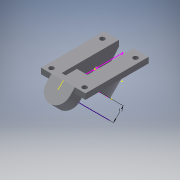
# Autodesk Inventor part: shaft_jig
Saved by Autodesk Inventor 2017 SP1 (Build 210196100, 196)
## iProperties
Part Number: shaft_jig
Material: 一般
Document SubType Name: Modeling
Designer: gisen
Density: 1 g/cm^3
Appearance: 既定
Author: gisen
Autodesk Inventor part; units mm, degrees
ref_plane "YZ Plane" through (0, 0, 0) normal (1, 0, 0) x (0, 1, 0)
ref_plane "XZ Plane" through (0, 0, 0) normal (0, 1, 0) x (-1, 0, 0)
ref_plane "XY Plane" through (0, 0, 0) normal (0, 0, 1) x (1, 0, 0)
sketch "スケッチ1" plane through (0, 0, 0) normal (0, 0, 1) x (1, 0, 0)
  line L0 (-27.5, -39) -> (27.5, -39)
  line L1 (27.5, -39) -> (27.5, 39)
  line L2 (27.5, 39) -> (-27.5, 39)
  line L3 (-27.5, 39) -> (-27.5, -39)
  line L4 (-27.5, -39) -> (27.5, 39) construction
  line L5 (27.5, -39) -> (-27.5, 39) construction
  point P0 (0, 0)
  dimension "d0" = 55
  dimension "d1" = 78
  constraints: 12 end point, 2 midpoint, 2 parallel, 1 horizontal, 1 perpendicular
  measures "d0" distance of L2.end L1.end
  measures "d1" distance of L1.end L0.end
extrude "押し出し1" add sketch "スケッチ1" along normal blind 7
sketch "スケッチ2" plane through (0, 0, 7) normal (0, 0, 1) x (1, 0, 0)
  line L0 (9, -27) -> (9, 39)
  line L1 (9, 39) -> (-9, 39)
  line L2 (-9, 39) -> (-9, -27)
  line L3 (-9, -27) -> (9, -27)
  line L4 (9, -27) -> (-9, 39) construction
  line L5 (9, 39) -> (-9, -27) construction
  point P0 (0, 0)
  point P1 (0, 6)
  dimension "d4" = 18
  dimension "d5" = 66
  dimension "d15" = 9
  constraints: 12 end point, 2 midpoint, 2 parallel, 1 perpendicular
  measures "d4" distance of L1.end L0.end
  measures "d5" distance of L0.start L0.end
  measures "d15" distance from line of L0 point (0, 0)
extrude "押し出し2" cut sketch "スケッチ2" against normal blind 7
ref_plane "作業平面1" through (-27.5, -39, 7) normal (0, 0.7071068, -0.7071068) x (1, 0, 0)
sketch "スケッチ5" plane through (-27.5, -39, 7) normal (0, 0.7071068, -0.7071068) x (1, 0, 0)
  line L0 (0, 4.9497) -> (55, 4.9497) projected
  line L1 (55, 4.9497) -> (55, 0) projected
  line L2 (0, 0) -> (55, 0) projected
  line L3 (0, 4.9497) -> (0, 0) projected
  line L4 (27.5, 9) -> (42, 9) construction
  line L5 (27.5, 9) -> (42, 9) construction
  line L6 (27.5, 9) -> (13, 9) construction
  line L7 (42, 0) -> (13, 0)
  line L8 (13, 0) -> (13, 9)
  line L9 (42, 9) -> (42, 0)
  line L10 (42, 9) -> (13, 9)
  line L11 (13, 9) -> (13, 0)
  line L12 (13, 0) -> (42, 0)
  line L13 (42, 0) -> (42, 9)
  arc A0 (42, 9) -> (13, 9) centre (27.5, 9) ccw
  point P0 (27.5, -22.6274)
  dimension "d14" = 180
  dimension "d16" = 9
  dimension "d17" = 0
  dimension "d18" = 9
  dimension "d19" = 55
  dimension "d20" = 27.5
  constraints: 20 end point, 2 horizontal, 2 parallel, 2 perpendicular, 2 point on circle, 1 centre point, 1 coincident, 1 collinear, 1 vertical
  measures "d14" angle of L6 L4
  measures "d16" distance of L5.end L7.start
  measures "d17" distance between parallel lines of L7 L2
  measures "d18" distance of L7.end L6.end
  measures "d19" distance of L0.start L0.end
  measures "d20" distance from line of L3 L4.start
extrude "押し出し4" add sketch "スケッチ5" along normal blind 17 contours L8 L10 L9 L0 | L0 L9 L2 L8 | A0 L10
sketch "スケッチ6" plane through (-14.5, -26.9792, -5.0208) normal (0, 0.7071068, 0.7071068) x (1, 0, 0)
  line L0 (5.5, -7.1005) -> (23.5, -7.1005) projected
  line L1 (29, -7.1005) -> (0, -7.1005) projected
  line L2 (29, -7.1005) -> (29, 0) projected
  line L3 (0, 0) -> (29, 0) projected
  line L4 (0, -7.1005) -> (0, 0) projected
  line L5 (0, -17) -> (0, 0) projected
  line L6 (29, -7.1005) -> (0, -7.1005)
  line L7 (0, -7.1005) -> (0, 0)
  line L8 (0, 0) -> (29, 0)
  line L9 (29, 0) -> (29, -7.1005)
  point P0 (14.5, 15.5269)
  constraints: 8 end point, 2 parallel, 1 horizontal, 1 perpendicular
extrude "押し出し5" add sketch "スケッチ6" along normal up to surface surface through (0, 0, 0) normal (0, 0, 1)
chamfer "面取り1" distance 5 angle 45 1 edges at (0, -27, 7)
sketch "スケッチ8" plane through (-9, -21.9584, 0) normal (0, 0, 1) x (1, 0, 0)
  line L0 (18, -5.0416) -> (18, 0) projected
  line L1 (0, 0) -> (18, 0) projected
  line L2 (0, 0) -> (0, -5.0416) projected
  line L3 (0, -5.0416) -> (18, -5.0416) projected
  line L4 (0, -5.0416) -> (18, -5.0416) projected
  line L5 (0, -5.0416) -> (18, -5.0416)
  line L6 (18, -5.0416) -> (18, 8.9584)
  line L7 (18, 8.9584) -> (0, 8.9584)
  line L8 (0, 8.9584) -> (0, -5.0416)
  point P0 (9, 21.9584)
  dimension "d30" = 14
  constraints: 8 end point, 2 parallel, 1 horizontal, 1 perpendicular
  measures "d30" distance of L6.end L5.end
extrude "押し出し8" add sketch "スケッチ8" along normal blind 2
ref_plane "作業平面2" through (-27.5, 1.3051, -33.3051) normal (0, 0.7071068, -0.7071068) x (-1, 0, 0)
ref_plane "作業平面3" through (7.25, -21.9584, 0) normal (0, 0.7071068, 0.7071068) x (1, 0, 0)
sketch "スケッチ9" plane through (7.25, -21.9584, 0) normal (0, 0.7071068, 0.7071068) x (1, 0, 0)
  line L0 (-21.75, 0) -> (-21.75, -12.0503) projected
  line L1 (-34.75, -12.0503) -> (-21.75, -12.0503) projected
  line L2 (-34.75, 43.1041) -> (-34.75, -12.0503) projected
  line L3 (-16.25, 43.1041) -> (-34.75, 43.1041) projected
  line L4 (-16.25, 43.1041) -> (-16.25, 6.3345) projected
  line L5 (1.75, 6.3345) -> (-16.25, 6.3345) construction
  line L6 (1.75, 6.3345) -> (1.75, 43.1041) projected
  line L7 (20.25, 43.1041) -> (1.75, 43.1041) projected
  line L8 (20.25, -12.0503) -> (20.25, 43.1041) projected
  line L9 (7.25, -12.0503) -> (20.25, -12.0503) projected
  line L10 (7.25, -12.0503) -> (7.25, 0) projected
  line L11 (-21.75, 0) -> (7.25, 0) projected
  line L12 (-7.25, 40) -> (7.75, 40) construction
  line L13 (-7.25, 40) -> (7.75, 40) construction
  line L14 (-7.25, 40) -> (-7.25, 51.8983) construction
  line L15 (7.25, 0) -> (-21.75, 0) projected
  line L16 (7.75, 40) -> (7.75, 0)
  line L17 (7.75, 0) -> (-22.25, 0)
  line L18 (-22.25, 0) -> (7.75, 0)
  circle A0 centre (-7.25, 40) radius 4.5 projected
  circle A1 centre (-7.25, 40) radius 11 projected
  spline S0 degree 2 poles (-7.25, 50) (-26.3864, 48.3359) (-22.25, 0) knots 0 0 0 1 1 1
  line L19 (-7.25, 40) -> (-7.25, 50)
  spline S1 degree 2 poles (-7.25, 50) (11.8864, 48.3359) (7.75, 0) knots 0 0 0 1 1 1
  point P0 (-7.25, 15.5269)
  point P1 (-17.8029, 43.1041)
  point P2 (3.3029, 43.1041)
  dimension "d103" = 15
  dimension "d106" = 10
  constraints: 14 end point, 3 point on line, 2 coincident, 2 collinear, 1 horizontal, 1 perpendicular, 1 symmetric about line, 1 vertical, 8 other
  measures "d103" distance from line of L16 L12.start
  measures "d106" distance of L12.start L19.end
extrude "押し出し9" add sketch "スケッチ9" along normal up to surface contours L17 S0 A1 S1 L16 L11 | L16 S1 | S0 S1 L7 L6 A1 L4 L3 | L3 L4 A1 | A1 L6 L7 surface through (0, 0, 0) normal (0, 0, 1)
ref_plane "作業平面4" through (9, -13, 2) normal (0, 0.7071068, 0.7071068) x (-1, 0, 0)
sketch "スケッチ13" plane through (0, 0, 0) normal (1, 0, 0) x (0, 1, 0)
  line L0 (39, 0) -> (39, 7) projected
  line L1 (39, 0) -> (26.8843, -21.868)
  line L2 (39, 0) -> (39, 7) projected
  line L3 (39, 0) -> (48.7906, 0)
  line L4 (40.9741, 0) -> (28.2462, 0) projected
  line L5 (39, 0) -> (48.7523, 0) projected
  line L6 (13.397, -35.3553) -> (48.7523, 0) construction
  line L7 (13.397, -35.3553) -> (8.5208, -30.4792) projected
  line L8 (8.5208, -30.4792) -> (39, 0) projected
  line L9 (39, 0) -> (-21.9584, 0) projected
  line L10 (8.5208, -30.4792) -> (-21.9584, 0) projected
  line L11 (48.7523, 0) -> (26.8843, -21.868)
  line L12 (39, 0) -> (26.8843, -21.868)
  line L13 (39, 0) -> (48.7523, 0)
  line L14 (26.8843, -21.868) -> (48.7523, 0)
  line L15 (13.397, -35.3553) -> (48.7523, 0) projected
  point P0 (0, 0)
  dimension "d107" = 25
  constraints: 12 end point, 3 collinear, 2 point on line
  measures "d107" distance of L0.start L1.end
ref_plane "作業平面5" through (27.5, 39, 7) normal (0, 0.7071068, 0.7071068) x (-1, 0, 0)
sketch "スケッチ16" plane through (27.5, 39, 7) normal (0, 0.7071068, 0.7071068) x (-1, 0, 0)
  line L0 (18.5, 33.234) -> (18.5, 43.1335) projected
  line L1 (18.5, 33.234) -> (36.5, 33.234)
  line L2 (36.5, 33.234) -> (36.5, -26.766)
  line L3 (36.5, -26.766) -> (18.5, -26.766)
  line L4 (18.5, -26.766) -> (18.5, 33.234)
  point P0 (27.5, 22.6274)
  dimension "d56" = 18
  dimension "d57" = 60
  constraints: 8 end point, 2 parallel, 1 horizontal, 1 perpendicular
  measures "d56" distance of L2.end L3.end
  measures "d57" distance of L1.end L2.end
extrude "押し出し13" cut sketch "スケッチ16" against normal blind 30
sketch "スケッチ17" plane through (9, -13, 2) normal (0, 0.7071068, 0.7071068) x (-1, 0, 0)
  line L0 (0, 0) -> (18, 0) projected
  line L1 (0, 0) -> (18, 0)
  line L2 (18, 0) -> (18, -12)
  line L3 (18, -12) -> (0, -12)
  line L4 (0, -12) -> (0, 0)
  point P0 (9, -10.6066)
  dimension "d60" = 18
  dimension "d61" = 12
  constraints: 8 end point, 2 parallel, 1 horizontal, 1 perpendicular
  measures "d60" distance of L2.end L3.end
  measures "d61" distance of L1.end L2.end
extrude "押し出し15" add sketch "スケッチ17" against normal blind 5
ref_plane "作業平面6" through (7.25, -12.0589, 9.8995) normal (0, -0.7071068, -0.7071068) x (-1, 0, 0)
ref_plane "作業平面8" through (-15, -28.9584, -7) normal (-1, 0, 0) x (0, 0, 1)
sketch "スケッチ22" plane through (-15, -28.9584, -7) normal (-1, 0, 0) x (0, 0, 1)
  line L0 (-21.2843, 35.2843) -> (7, 63.5685) projected
  line L1 (-21.2843, 35.2843) -> (0, 14) projected
  line L2 (0, -0.8048) -> (0, 14) projected
  line L3 (7, 63.5685) -> (7, 31.0416) projected
  line L4 (-21.2843, 35.2843) -> (0, 14) projected
  line L5 (-2.8995, 16.8995) -> (7, 26.799)
  line L6 (9, 15.9584) -> (-4.435, 29.3934) projected
  line L7 (-2.8995, 16.8995) -> (11.1005, 16.8995) construction
  line L8 (7, 67.9584) -> (7, -10.0416) projected
  line L9 (-2.8259, 40.8675) -> (7, 31.0416) projected
  line L10 (7, 26.799) -> (-4.9472, 38.7462) projected
  line L11 (-4.9472, 38.7462) -> (-2.8259, 40.8675) projected
  line L12 (7, -0.8048) -> (0, -0.8048) projected
  line L13 (7, 26.799) -> (7, -0.8048) projected
  point P0 (7, 28.9584)
  point P1 (7, 7)
  dimension "d81" = 14
  dimension "d82" = 45
  constraints: 4 end point, 2 point on line, 1 coincident, 1 equal length, 1 horizontal, 1 perpendicular
  measures "d81" distance of L5.start L5.end
  measures "d82" angle of L7 L5
sketch "スケッチ24" plane through (0, 0, 0) normal (1, 0, 0) x (0, 1, 0)
  line L0 (-45.364, 0.636) -> (-45.364, 0.636) projected
  line L1 (-45.364, 0.636) -> (-33.3431, -11.3848) projected
  line L2 (-33.3431, -11.3848) -> (-33.3431, -11.3848) projected
  line L3 (-45.364, 0.636) -> (-33.3431, -11.3848) projected
  line L4 (-39, 7) -> (-39, 0) projected
  line L5 (-39, 7) -> (-45.364, 0.636) projected
  line L6 (-45.364, 0.636) -> (-33.3431, -11.3848) projected
  line L7 (-33.3431, -11.3848) -> (-21.9584, 0) projected
  line L8 (-39, 0) -> (-21.9584, 0) projected
  line L9 (9.7878, -11.9472) -> (-2.1594, 0) projected
  line L10 (-29.7632, 0) -> (-2.1594, 0) projected
  line L11 (-29.7632, -7) -> (-14.9584, -7) projected
  line L12 (-14.9584, -7) -> (6.3259, -28.2843) projected
  line L13 (6.3259, -28.2843) -> (34.6102, 0) projected
  line L14 (2.0833, 0) -> (11.9092, -9.8259) projected
  line L15 (11.9092, -9.8259) -> (9.7878, -11.9472) projected
  line L16 (26.1289, -22.5553) -> (28.38, -24.8064) projected
  line L17 (13.3629, -35.3213) -> (16.6424, -38.6008) projected
  line L18 (-33.9792, -12.0208) -> (18.1689, -64.1689)
  line L19 (6.3259, -28.2843) -> (-14.9584, -7) projected
  line L20 (26.8402, -28.4029) -> (16.6424, -38.6008) projected
  line L21 (28.38, -24.8064) -> (26.8402, -28.4029) projected
  line L22 (13.3629, -35.3213) -> (26.1289, -22.5553) projected
  line L23 (16.6424, -38.6008) -> (13.3629, -35.3213) projected
  line L24 (16.6424, -38.6008) -> (26.8402, -28.4029) projected
  line L25 (26.1289, -22.5553) -> (13.3629, -35.3213) projected
  line L26 (28.38, -24.8064) -> (26.1289, -22.5553) projected
  line L27 (26.8402, -28.4029) -> (28.38, -24.8064) projected
  line L28 (-29.7632, 0) -> (-29.7632, -7) projected
  line L29 (2.0833, 0) -> (34.6102, 0) projected
  point P0 (0, 0)
  point P1 (28.1075, -24.5339)
  point P2 (33.7643, -30.1908)
  point P3 (20.9984, -42.9567)
  point P4 (15.3415, -37.2999)
  dimension "d93" = 17
  constraints: 2 end point, 1 coincident, 1 parallel
  measures "d93" distance between parallel lines of L12 L18
sketch "スケッチ25" plane through (-27.5, -26.9792, -5.0208) normal (0, 0.7071068, -0.7071068) x (-1, 0, 0)
  circle A0 centre (-27.5, -9.8995) radius 4
  point P0 (-27.5, 22.6274)
  point P1 (-27.5, -9)
  dimension "d94" = 8
  constraints: 2 coincident, 1 centre point
  measures "d94" diameter of A0
extrude "押し出し21" cut sketch "スケッチ25" against normal blind 10
thread "ねじ3" size "M8x1.25" class "6H" standard "ANSI Metric M Profile" full length
extrude "押し出し23" cut sketch "スケッチ13" along normal through all both and the other way through all contours L3 L11 L1
sketch "スケッチ29" plane through (0, 0, 0) normal (1, 0, 0) x (0, 1, 0)
  line L0 (39, 0) -> (35.1747, -6.9045) projected
  line L1 (35.1747, -6.9045) -> (22.8264, -19.2528) projected
  line L2 (22.8264, -19.2528) -> (26.163, -22.5894) projected
  line L3 (13.397, -35.3553) -> (26.163, -22.5894) projected
  line L4 (13.397, -35.3553) -> (8.5208, -30.4792) projected
  line L5 (8.5208, -30.4792) -> (39, 0) projected
  line L6 (39, 0) -> (-21.9584, 0) projected
  line L7 (8.5208, -30.4792) -> (-21.9584, 0) projected
  line L8 (39, 0) -> (39, 7) projected
  line L9 (22.8264, -19.2528) -> (39, 0)
  line L10 (39, 0) -> (38.365, -14.2549)
  line L11 (38.365, -14.2549) -> (22.8264, -19.2528)
  point P0 (0, 0)
  constraints: 6 end point
extrude "押し出し25" cut sketch "スケッチ29" along normal through all both and the other way through all contours L0 L1 L9
sketch "スケッチ30" plane through (27.5, 17.7868, -14.2132) normal (0, 0.7071068, 0.7071068) x (1, 0, 0)
  circle A0 centre (-27.5, 1.8457) radius 4.5 projected
  line L0 (-36.5, -20.1005) -> (-36.5, 7.127) projected
  line L1 (-18.5, -20.1005) -> (-36.5, -20.1005) projected
  line L2 (-18.5, 7.127) -> (-18.5, -20.1005) projected
  arc A1 (-18.5, -10.3909) -> (-36.5, -10.3909) centre (-27.5, -28.2262) ccw
  line L3 (-27.5, -8.2487) -> (-27.5, -28.2487)
  arc A2 (-34.5711, -25.3198) -> (-27.5, -28.2487) centre (-27.5, -18.2487) ccw
  line L4 (-27.5, -18.2487) -> (-34.5711, -25.3198) construction
  line L5 (-27.5, -18.2487) -> (-27.5, -28.2487) construction
  arc A3 (-27.5, -28.2487) -> (-20.4289, -25.3198) centre (-27.5, -18.2487) ccw
  line L6 (-27.5, -18.2487) -> (-20.4289, -25.3198) construction
  line L7 (-27.5, -18.2487) -> (-27.5, -28.2487) construction
  line L8 (-36.5, -10.3909) -> (-36.5, -23.3909)
  line L9 (-36.5, -50.2046) -> (-36.5, 0) projected
  line L10 (-36.5, -23.3909) -> (-34.5711, -25.3198)
  line L11 (-18.5, -10.3909) -> (-18.5, -23.3909)
  line L12 (-18.5, -23.3909) -> (-20.4289, -25.3198)
  point P0 (-27.5, -22.6274)
  dimension "d123" = 20
  dimension "d124" = 45
  dimension "d125" = 45
  dimension "d126" = 13
  constraints: 18 end point, 7 point on circle, 3 centre point, 3 point on line, 1 coincident, 1 midpoint, 1 perpendicular, 1 symmetric about line, 1 vertical, 2 other
  measures "d123" distance of L3.start L3.end
  measures "d124" angle of L4 L5
  measures "d125" angle of L7 L6
  measures "d126" distance of L8.start L8.end
extrude "押し出し26" cut sketch "スケッチ30" against normal through all contours L0 A1 L3 L1 | L1 L3 A2 L10 L8 | L3 A1 L2 L1 | L1 L11 L12 A3 L3
sketch "スケッチ31" plane through (9, -13, 2) normal (0, 0.7071068, 0.7071068) x (1, 0, 0)
  line L0 (0, 0) -> (-18, 0) projected
  line L1 (-18, 22.8431) -> (-18, 9.8431) projected
  line L2 (0, 0) -> (-18, 0)
  line L3 (-18, 0) -> (-18, 13)
  line L4 (-18, 13) -> (0, 13)
  line L5 (0, 13) -> (0, 0)
  point P0 (-9, 10.6066)
  dimension "d129" = 13
  constraints: 8 end point, 2 parallel, 1 horizontal, 1 perpendicular, 1 point on line
  measures "d129" distance of L2.end L3.end
extrude "押し出し27" cut sketch "スケッチ31" along normal through all
sketch "スケッチ32" plane through (0, 0, 7) normal (0, 0, 1) x (1, 0, 0)
  line L0 (27.5, -39) -> (27.5, 39) projected
  line L1 (9, 39) -> (9, -32) projected
  line L2 (-9, -32) -> (-9, 39) projected
  line L3 (-9, 39) -> (-27.5, 39) projected
  line L4 (-27.5, 39) -> (-27.5, -39) projected
  line L5 (-27.5, -39) -> (-14.5, -39) projected
  line L6 (-14.5, -39) -> (14.5, -39) projected
  line L7 (14.5, -39) -> (27.5, -39) projected
  line L8 (27.5, -39) -> (27.5, 39) projected
  line L9 (27.5, 39) -> (9, 39) projected
  line L10 (9, 39) -> (9, -32) projected
  line L11 (-9, -32) -> (9, -32) projected
  line L12 (0, 0) -> (0, -32)
  point P0 (20.5, 30)
  point P1 (20.5, -33)
  point P2 (-20.5, 30)
  point P3 (-20.5, -33)
  dimension "d132" = 9
  dimension "d133" = 7
  dimension "d134" = 6
  dimension "d135" = 7
  constraints: 2 end point, 2 symmetric about line, 1 midpoint
  measures "d132" distance from line of point (20.5, 30) L9
  measures "d133" distance from line of point (20.5, 30) L0
  measures "d134" distance from line of L7 point (20.5, -33)
  measures "d135" distance from line of L0 point (20.5, -33)
hole "穴1" at (20.5, 30, 7) at (20.5, -33, 7) at (-20.5, -33, 7) at (-20.5, 30, 7) direction (0, 0, -1) diameter 6 end through all
equation "\"d15\" = 0.5 * d4"
equation "\"d20\" = 0.5 * d19"
